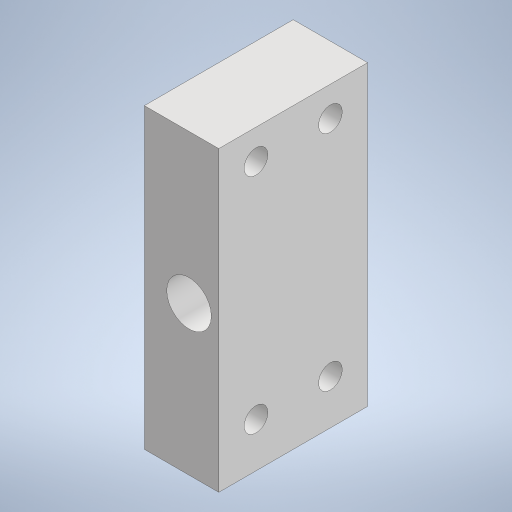
# Autodesk Inventor part: z_shaft_block
Saved by Autodesk Inventor 2024.1 (Build 281209000, 209)
## iProperties
Created: 2023-10-06
Part Number: z_shaft_block
Material: Generic
Document SubType Name: Modeling
Designer: l1534
Density: 1 g/cm^3
Appearance: Default
Author: l1534
Autodesk Inventor part; units mm, degrees
ref_plane "YZ Plane" through (0, 0, 0) normal (1, 0, 0) x (0, 1, 0)
ref_plane "XZ Plane" through (0, 0, 0) normal (0, 1, 0) x (-1, 0, 0)
ref_plane "XY Plane" through (0, 0, 0) normal (0, 0, 1) x (1, 0, 0)
sketch "Sketch1" plane through (0, 0, 0) normal (1, 0, 0) x (0, 1, 0)
  line L0 (-9.5937, 6.5342) -> (10.4063, 6.5342)
  line L1 (10.4063, 6.5342) -> (10.4063, -3.4658)
  line L2 (10.4063, -3.4658) -> (-9.5937, -3.4658)
  line L3 (-9.5937, -3.4658) -> (-9.5937, 6.5342)
  point P0 (0, 0)
  dimension "d0" = 20
  dimension "d1" = 10
  constraints: 8 end point, 2 parallel, 1 horizontal, 1 perpendicular
  measures "d0" distance of L0.start L0.end
  measures "d1" distance of L0.end L1.end
extrude "Extrusion1" add sketch "Sketch1" along normal blind 5
sketch "Sketch2" plane through (0, -9.5937, 6.5342) normal (0, 0, 1) x (1, 0, 0)
  circle A0 centre (3, 10) radius 1.5
  line L0 (5, 20) -> (5, 0) projected
  line L1 (0, 20) -> (5, 20) projected
  point P0 (0, 9.5937)
  dimension "d4" = 3
  dimension "d5" = 2
  dimension "d6" = 10
  constraints: 1 centre point
  measures "d4" diameter of A0
  measures "d5" distance from line of L0 A0.centre
  measures "d6" distance from line of L1 A0.centre
extrude "Extrusion2" cut sketch "Sketch2" against normal through all
sketch "Sketch3" plane through (5, 0, 0) normal (1, 0, 0) x (0, 0, -1)
  circle A0 centre (-4.0342, -6.5937) radius 0.8
  circle A1 centre (0.9658, -6.5937) radius 0.8
  circle A2 centre (-4.0342, 8.4063) radius 0.8
  circle A3 centre (0.9658, 8.4063) radius 0.8
  line L0 (-6.5342, 10.4063) -> (-6.5342, -9.5937) projected
  line L1 (3.4658, -9.5937) -> (3.4658, 10.4063) projected
  line L2 (-6.5342, -9.5937) -> (3.4658, -9.5937) projected
  point P0 (0, 0)
  dimension "d9" = 1.6
  dimension "d11" = 1.6
  dimension "d12" = 1.6
  dimension "d13" = 1.6
  dimension "d14" = 2.5
  dimension "d15" = 2.5
  dimension "d16" = 3
  dimension "d17" = 3
  dimension "d18" = 15
  dimension "d19" = 15
  dimension "d20" = 2.5
  dimension "d21" = 2.5
  constraints: 4 centre point
  measures "d9" diameter of A0
  measures "d11" diameter of A2
  measures "d12" diameter of A3
  measures "d13" diameter of A1
  measures "d14" distance from line of L0 A0.centre
  measures "d15" distance from line of L1 A1.centre
  measures "d16" distance from line of L2 A0.centre
  measures "d17" distance from line of L2 A1.centre
  measures "d18" distance of A2.centre A0.centre
  measures "d19" distance of A1.centre A3.centre
  measures "d20" distance from line of L1 A3.centre
  measures "d21" distance from line of L0 A2.centre
extrude "Extrusion3" cut sketch "Sketch3" against normal through all
body "Solid1"
